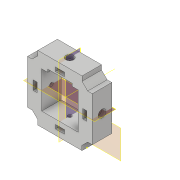
# Autodesk Inventor part: 30_Cube_Z_Focus_MGN_NEMA_Motorsupport_centered
Saved by Autodesk Inventor 2022 (Build 260153000, 153)
## iProperties
Created: 2019-07-01
Part Number: 30_Cube_Z_Focus_MGN_NEMA_Motorsupport_centered
Material: Generic
Document SubType Name: Modeling
Designer: diederichbenedict
Density: 1 g/cm^3
Appearance: Default
Author: diederichbenedict
Autodesk Inventor part; units mm, degrees
ref_plane "YZ Plane" through (0, 0, 0) normal (1, 0, 0) x (0, 1, 0)
ref_plane "XZ Plane" through (0, 0, 0) normal (0, 1, 0) x (-1, 0, 0)
ref_plane "XY Plane" through (0, 0, 0) normal (0, 0, 1) x (1, 0, 0)
ref_plane "Work Plane5" through (0, 0, 10) normal (0, 0, 1) x (1, 0, 0)
sketch "Sketch1" plane through (0, 0, 10) normal (0, 0, 1) x (1, 0, 0)
  line L0 (-4.0299, -0.3538) -> (-2.2322, 1.4439) construction
  arc A0 (-1.4439, 2.2322) -> (-2.2322, 1.4439) centre (-0.9299, 0.9299) ccw construction
  line L1 (-1.4439, 2.2322) -> (0.3538, 4.0299) construction
  line L2 (-37.8299, 42.8299) -> (-37.8299, 37.8299) construction
  line L3 (-37.8299, 37.8299) -> (-42.9208, 37.8299) construction
  line L4 (-37.8299, 42.2137) -> (-37.8299, 45.8299) construction
  line L5 (-37.8299, 45.8299) -> (-4.0299, 45.8299) construction
  line L6 (-4.0299, 45.8299) -> (-4.0299, 42.2137) construction
  line L7 (-4.0299, 4.0299) -> (0.3538, 4.0299) projected
  circle A1 centre (-20.9299, 20.9299) radius 17.5 projected
  line L8 (-20.9299, 58.9723) -> (17.1124, 20.9299) construction
  line L9 (17.1124, 20.9299) -> (-20.9299, -17.1124) construction
  line L10 (-20.9299, -17.1124) -> (-58.9723, 20.9299) construction
  line L11 (-58.9723, 20.9299) -> (-20.9299, 58.9723) construction
  line L12 (-20.9299, 58.9723) -> (-20.9299, -17.1124) construction
  line L13 (17.1124, 20.9299) -> (-58.9723, 20.9299) construction
  line L14 (-20.9299, 58.9723) -> (32.8701, 58.9723) construction
  line L15 (-43.4299, 43.4299) -> (1.5701, 43.4299) construction
  line L16 (1.5701, 43.4299) -> (1.5701, -1.5701) construction
  line L17 (1.5701, -1.5701) -> (-43.4299, -1.5701) construction
  line L18 (-43.4299, -1.5701) -> (-43.4299, 43.4299) construction
  line L19 (-43.4299, 43.4299) -> (1.5701, -1.5701) construction
  line L20 (1.5701, 43.4299) -> (-43.4299, -1.5701) construction
  line L21 (-43.4299, 5.3876) -> (-43.4299, 36.4723)
  line L22 (-43.4299, 36.4723) -> (-36.4723, 43.4299)
  line L23 (-36.4723, 43.4299) -> (-5.3876, 43.4299)
  line L24 (-5.3876, 43.4299) -> (1.5701, 36.4723)
  line L25 (1.5701, 36.4723) -> (1.5701, 5.3876)
  line L26 (1.5701, 5.3876) -> (-5.3876, -1.5701)
  line L27 (-5.3876, -1.5701) -> (-36.4723, -1.5701)
  line L28 (-36.4723, -1.5701) -> (-43.4299, 5.3876)
  line L29 (-4.0299, 42.2137) -> (-37.8299, 42.2137) projected
  line L30 (-4.0299, -0.3538) -> (-4.0299, 4.0299) projected
  circle A2 centre (-20.9299, 20.9299) radius 1.5
  line L31 (-10.9299, 10.9299) -> (-30.9299, 10.9299) construction
  line L32 (-30.9299, 10.9299) -> (-30.9299, 30.9299) construction
  line L33 (-30.9299, 30.9299) -> (-10.9299, 30.9299) construction
  line L34 (-10.9299, 30.9299) -> (-10.9299, 10.9299) construction
  line L35 (-10.9299, 10.9299) -> (-30.9299, 30.9299) construction
  line L36 (-30.9299, 10.9299) -> (-10.9299, 30.9299) construction
  circle A3 centre (-30.9299, 30.9299) radius 1.4
  circle A4 centre (-30.9299, 10.9299) radius 1.4
  circle A5 centre (-10.9299, 10.9299) radius 1.4
  line L37 (-45.8299, 37.8299) -> (-42.0723, 37.8299) construction
  line L38 (-42.1723, 37.7299) -> (-45.8299, 37.7299)
  line L39 (-45.8299, 37.7299) -> (-45.8299, 4.1299)
  line L40 (-45.8299, 4.1299) -> (-42.1723, 4.1299)
  line L41 (-42.1723, 4.1299) -> (-42.1723, 37.7299)
  line L42 (-45.8299, 4.0299) -> (-42.0723, 4.0299) construction
  line L43 (-45.8299, 37.8299) -> (-42.0723, 37.8299) projected
  line L44 (-37.7299, 45.8299) -> (-4.1299, 45.8299)
  line L45 (-4.1299, 45.8299) -> (-4.1299, 42.1723)
  line L46 (-4.1299, 42.1723) -> (-37.7299, 42.1723)
  line L47 (-37.7299, 42.1723) -> (-37.7299, 45.8299)
  line L48 (0.4701, 37.8299) -> (0.4701, 4.0299) construction
  line L49 (0.4701, 4.0299) -> (3.9701, 4.0299) construction
  line L50 (3.9701, 37.8299) -> (3.9701, 4.0299) construction
  line L51 (0.4701, 37.8299) -> (3.9701, 37.8299) construction
  line L52 (-45.8299, -3.9701) -> (-4.0299, -3.9701) construction
  line L53 (0.3124, 37.7299) -> (3.9701, 37.7299)
  line L54 (3.9701, 37.7299) -> (3.9701, 4.1299)
  line L55 (3.9701, 4.1299) -> (0.3124, 4.1299)
  line L56 (0.3124, 4.1299) -> (0.3124, 37.7299)
  line L57 (-4.1713, -0.3538) -> (-37.7299, -0.3538)
  line L58 (-37.7299, -0.3538) -> (-37.7299, -3.9701)
  line L59 (-37.7299, -3.9701) -> (-4.1713, -3.9701)
  line L60 (-4.1713, -3.9701) -> (-4.1713, -0.3538)
  point P0 (-37.8299, 4.0299)
  dimension "d18" = 53.8
  dimension "d19" = 45
  dimension "d20" = 53.8
  dimension "d21" = 45
  dimension "d22" = 45
  dimension "d30" = 20
  dimension "d31" = 20
  dimension "d32" = 2.8
  dimension "d33" = 2.8
  dimension "d34" = 2.8
  dimension "d35" = 3
  dimension "d36" = 0.1
  dimension "d37" = 0.1
  dimension "d38" = 0.1
  dimension "d39" = 0.1
  constraints: 86 end point, 21 point on line, 14 parallel, 8 perpendicular, 7 horizontal, 7 midpoint, 4 centre point, 4 coincident, 1 equal length
  measures "d18" distance of L8.start L8.end
  measures "d19" angle of L8 L14
  measures "d20" distance of L8.end L9.end
  measures "d21" distance of L16.end L17.end
  measures "d22" distance of L15.end L16.end
  measures "d30" distance of L32.end L33.end
  measures "d31" distance of L31.end L32.end
  measures "d32" diameter of A3
  measures "d33" diameter of A4
  measures "d34" diameter of A5
  measures "d35" diameter of A2
  measures "d36" distance between parallel lines of L38 L43
  measures "d37" distance between parallel lines of L40 L42
  measures "d38" distance between parallel lines of L45 L6
  measures "d39" distance between parallel lines of L4 L47
extrude "Extrusion1" add sketch "Sketch1" along normal blind 15 contours L30 L26 L57 L28 L41 L22 L46 L24 L56 L7 | L7 L26 L30 | L56 L24 L25 L26 | L26 L25 L24 L53 L54 L55 | L60 L59 L58 L57 L28 L27 L26 | L26 L27 L28 L57 | L46 L22 L29 L24 | L24 L29 L45 | L40 L39 L38 L22 L21 L28 | L28 L21 L22 L41 | L29 L22 L23 L24 | L24 L23 L22 L29 L47 L44 L45 | L47 L29 L22 | A1 | A2 | A3 | A4 | A5
sketch "Skizze4" plane through (0, 0, 25) normal (0, 0, 1) x (1, 0, 0)
  line L0 (-37.7299, 42.1723) -> (-42.1723, 37.7299) projected
  line L1 (-42.1723, 37.7299) -> (-45.8299, 37.7299) projected
  line L2 (-45.8299, 37.7299) -> (-45.8299, 4.1299) construction
  line L3 (-45.8299, 4.1299) -> (-42.1723, 4.1299) projected
  line L4 (-42.1723, 4.1299) -> (-37.6885, -0.3538) projected
  line L5 (-37.6885, -0.3538) -> (-37.7299, -0.3538) projected
  line L6 (-37.7299, -0.3538) -> (-37.7299, -3.9701) projected
  line L7 (-37.7299, -3.9701) -> (-4.1713, -3.9701) construction
  line L8 (-4.1713, -3.9701) -> (-4.1713, -0.3538) projected
  line L9 (-4.1713, -0.3538) -> (0.3124, 4.1299) projected
  line L10 (0.3124, 4.1299) -> (3.9701, 4.1299) projected
  line L11 (3.9701, 4.1299) -> (3.9701, 37.7299) construction
  line L12 (3.9701, 37.7299) -> (0.3124, 37.7299) projected
  line L13 (0.3124, 37.7299) -> (-4.1299, 42.1723) projected
  line L14 (-4.1299, 42.1723) -> (-4.1299, 45.8299) projected
  line L15 (-4.1299, 45.8299) -> (-37.7299, 45.8299) construction
  line L16 (-37.7299, 45.8299) -> (-37.7299, 42.1723) projected
  line L17 (-37.9299, 46.0299) -> (-3.9299, 46.0299) construction
  line L18 (-3.9299, 46.0299) -> (-3.9299, 42.2551)
  line L19 (-3.9299, 42.2551) -> (0.3953, 37.9299)
  line L20 (0.3953, 37.9299) -> (4.1701, 37.9299)
  line L21 (4.1701, 37.9299) -> (4.1701, 3.9299) construction
  line L22 (4.1701, 3.9299) -> (0.3953, 3.9299)
  line L23 (0.3953, 3.9299) -> (-3.9713, -0.4367)
  line L24 (-3.9713, -0.4367) -> (-3.9713, -4.1701)
  line L25 (-3.9713, -4.1701) -> (-37.9299, -4.1701) construction
  line L26 (-37.9299, -4.1701) -> (-37.9299, -0.3953)
  line L27 (-37.9299, -0.3953) -> (-42.2551, 3.9299)
  line L28 (-42.2551, 3.9299) -> (-46.0299, 3.9299)
  line L29 (-46.0299, 3.9299) -> (-46.0299, 37.9299) construction
  line L30 (-46.0299, 37.9299) -> (-42.2551, 37.9299)
  line L31 (-42.2551, 37.9299) -> (-37.9299, 42.2551)
  line L32 (-37.9299, 42.2551) -> (-37.9299, 46.0299)
  line L33 (-45.8299, 37.7299) -> (-45.8299, 37.9299)
  line L34 (-4.1299, 45.8299) -> (-37.7299, 45.8299) projected
  line L35 (-37.7299, 45.8299) -> (-37.9299, 45.8299)
  line L36 (-4.1299, 45.8299) -> (-3.9299, 45.8299)
  line L37 (3.9701, 37.7299) -> (3.9701, 37.9299)
  line L38 (3.9701, 4.1299) -> (3.9701, 37.7299) projected
  line L39 (3.9701, 4.1299) -> (3.9701, 3.9299)
  line L40 (-4.1713, -3.9701) -> (-3.9713, -3.9701)
  line L41 (-37.7299, -3.9701) -> (-37.9299, -3.9701)
  line L42 (-45.8299, 4.1299) -> (-45.8299, 3.9299)
  point P0 (0, 0)
  dimension "d40" = 0.2
  constraints: 48 end point, 12 point on line, 4 perpendicular, 15 other
  measures "d40" distance between parallel lines of L15 L17
extrude "IM_offset" add sketch "Skizze4" against normal up to surface (15 mm away)
sketch "Sketch29" plane through (0, 0, 10) normal (0, 0, -1) x (-1, 0, 0)
  line L0 (30.9299, 15.9299) -> (30.9299, 25.9299)
  line L1 (25.9299, 30.9299) -> (15.8299, 30.9299)
  line L2 (10.9299, 29.4299) -> (10.9299, 12.4299)
  line L3 (29.4299, 10.9299) -> (12.4299, 10.9299)
  line L4 (10.9299, 10.9299) -> (30.9299, 10.9299) construction
  line L5 (30.9299, 10.9299) -> (30.9299, 30.9299)
  line L6 (30.9299, 30.9299) -> (10.9299, 30.9299)
  line L7 (10.9299, 30.9299) -> (10.9299, 10.9299)
  line L8 (10.8299, 10.8299) -> (31.0299, 10.8299)
  line L9 (31.0299, 10.8299) -> (31.0299, 31.0299)
  line L10 (31.0299, 31.0299) -> (10.8299, 31.0299)
  line L11 (10.8299, 31.0299) -> (10.8299, 10.8299)
  circle A0 centre (20.9299, 20.9299) radius 11
  line L12 (13.0299, 34.4299) -> (28.8299, 34.4299)
  line L13 (6.9299, 12.5299) -> (6.9299, 29.3299)
  line L14 (34.9299, 9.4299) -> (34.9299, 32.4299)
  line L15 (29.3299, 6.9299) -> (12.5299, 6.9299)
  line L16 (12.5299, 34.9299) -> (29.3299, 34.9299)
  line L17 (34.9299, 6.9299) -> (6.9299, 6.9299)
  line L18 (6.9299, 6.9299) -> (6.9299, 34.9299)
  line L19 (6.9299, 34.9299) -> (34.9299, 34.9299)
  line L20 (34.9299, 34.9299) -> (34.9299, 6.9299)
  line L21 (34.9299, 6.9299) -> (6.9299, 34.9299) construction
  line L22 (6.9299, 6.9299) -> (34.9299, 34.9299) construction
  line L23 (35.0299, 35.0299) -> (6.8299, 35.0299)
  line L24 (6.8299, 35.0299) -> (6.8299, 6.8299)
  line L25 (6.8299, 6.8299) -> (35.0299, 6.8299)
  line L26 (35.0299, 6.8299) -> (35.0299, 35.0299)
  point P0 (0, 0)
  dimension "d188" = 0.1
  dimension "d189" = 0.1
  constraints: 54 end point, 8 parallel, 7 horizontal, 4 perpendicular, 4 vertical, 2 midpoint, 1 centre point, 26 other
  measures "d188" distance between parallel lines of L7 L11
  measures "d189" distance between parallel lines of L19 L23
extrude "Extrusion23" cut sketch "Sketch29" against normal through all contours A0 L3 L2 L1 L0 | A0 L9 L8 | L0 A0 L9 | A0 L1 L6 L5 L0 | L0 L5 L6 L1 A0 L10 L9 | A0 L8 L3 | L9 A0 | L1 A0 L10 | A0 L8 L11 | A0 L8 | A0 L2 L7 L6 L1 | L1 L6 L7 L2 A0 L11 L10 | L10 A0 | A0 L11 L2 | A0 L11 | L13 L18 L19 L16 L20 L14 L17 L15 | L26 L25 L24 L23
sketch "Sketch30" plane through (-45.8299, 0, 10) normal (-1, 0, 0) x (0, 0, 1)
  line L0 (35.0799, 45.8299) -> (6.8799, 45.8299)
  line L1 (0, 3.9299) -> (0, 37.9299) projected
  line L2 (15, 3.9299) -> (0, 3.9299) projected
  line L3 (15, 37.9299) -> (15, 3.9299) projected
  line L4 (15, 37.9299) -> (0, 37.9299) projected
  circle A0 centre (7.5, 20.9299) radius 1.7201
  point P0 (-10, 0)
  constraints: 2 end point, 1 centre point, 1 horizontal
ref_plane "Arbeitsebene7" through (-20.9299, 3.9299, 10) normal (-1, 0, 0) x (0, 0, 1)
ref_plane "Arbeitsebene8" through (-37.9299, 20.9299, 10) normal (0, 1, 0) x (1, 0, 0)
ref_plane "Arbeitsebene9" through (-20.9299, 3.9299, 10) normal (-1, 0, 0) x (0, 0, 1)
ref_plane "Arbeitsebene10" through (-37.9299, 20.9299, 10) normal (0, -1, 0) x (1, 0, 0)
hole "Bohrung2" at (-45.8299, 20.9299, 17.5) direction (1, 0, 0) diameter 2.8 end through all counterbore diameter 6 counterbore depth 3
pattern_circular "Runde Anordnung2" count 4 over 360 about axis through (-20.9299, 20.9299, 10) along (0, 0, 1) of "Bohrung2"
ref_plane "Arbeitsebene11" through (-20.9299, 3.9299, 10) normal (1, 0, 0) x (0, 0, -1)
ref_plane "Arbeitsebene12" through (-37.9299, 20.9299, 10) normal (0, 1, 0) x (1, 0, 0)
sketch "Sketch31" plane through (0, 0, 25) normal (0, 0, 1) x (1, 0, 0)
  point P0 (0, 0)
sketch "Sketch32" plane through (0, 0, 25) normal (0, 0, 1) x (1, 0, 0)
  line L0 (-6.8299, 6.8299) -> (-35.0299, 6.8299) projected
  line L1 (-35.0299, 6.8299) -> (-35.0299, 35.0299) projected
  line L2 (-35.0299, 35.0299) -> (-6.8299, 35.0299) projected
  line L3 (-6.8299, 35.0299) -> (-6.8299, 6.8299) projected
  line L4 (3.9701, 3.9299) -> (3.9701, 37.9299) projected
  line L5 (3.9701, 37.9299) -> (0.3953, 37.9299) projected
  line L6 (0.3953, 37.9299) -> (-3.9299, 42.2551) projected
  line L7 (-3.9299, 42.2551) -> (-3.9299, 45.8299) projected
  line L8 (-3.9299, 45.8299) -> (-37.9299, 45.8299) projected
  line L9 (-37.9299, 45.8299) -> (-37.9299, 42.2551) projected
  line L10 (-37.9299, 42.2551) -> (-42.2551, 37.9299) projected
  line L11 (-42.2551, 37.9299) -> (-45.8299, 37.9299) projected
  line L12 (-45.8299, 37.9299) -> (-45.8299, 3.9299) projected
  line L13 (-42.2551, 3.9299) -> (-45.8299, 3.9299) projected
  line L14 (-37.9299, -0.3953) -> (-42.2551, 3.9299) projected
  line L15 (-37.9299, -3.9701) -> (-37.9299, -0.3953) projected
  line L16 (-3.9713, -3.9701) -> (-37.9299, -3.9701) projected
  line L17 (-3.9713, -3.9701) -> (-3.9713, -0.4367) projected
  line L18 (-3.9713, -0.4367) -> (0.3953, 3.9299) projected
  line L19 (0.3953, 3.9299) -> (3.9701, 3.9299) projected
  line L20 (-22.3299, 42.8299) -> (-22.3299, 35.0299) projected
  line L21 (-19.5299, 42.8299) -> (-19.5299, 35.0299) projected
  line L22 (0.9701, 22.3299) -> (-6.8299, 22.3299) projected
  line L23 (0.9701, 19.5299) -> (-6.8299, 19.5299) projected
  line L24 (-19.5299, 6.8299) -> (-19.5299, -0.9701) projected
  line L25 (-22.3299, 6.8299) -> (-22.3299, -0.9701) projected
  line L26 (-35.0299, 19.5299) -> (-42.8299, 19.5299) projected
  line L27 (-35.0299, 22.3299) -> (-42.8299, 22.3299) projected
  line L28 (-41.5925, 24.4299) -> (-38.5925, 24.4299)
  line L29 (-38.5925, 24.4299) -> (-38.5925, 17.4299)
  line L30 (-38.5925, 17.4299) -> (-41.5925, 17.4299)
  line L31 (-41.5925, 17.4299) -> (-41.5925, 24.4299)
  line L32 (-41.5925, 24.4299) -> (-38.5925, 17.4299) construction
  line L33 (-38.5925, 24.4299) -> (-41.5925, 17.4299) construction
  point P0 (0, 0)
  point P1 (-40.0925, 20.9299)
  dimension "d190" = 3
  dimension "d191" = 7
  constraints: 12 end point, 2 midpoint, 2 parallel, 1 horizontal, 1 perpendicular
  measures "d190" distance of L29.end L30.end
  measures "d191" distance of L28.end L29.end
extrude "Extrusion25" cut sketch "Sketch32" against normal through all contours L29 L30 L31 L26 | L26 L31 L27 L29 | L27 L31 L28 L29
pattern_circular "Circular Pattern3" count 4 over 360 about axis through (-20.9299, 20.9299, 10) along (0, 0, 1) of "Extrusion25"
sketch "Sketch33" plane through (0, 0, 25) normal (0, 0, 1) x (1, 0, 0)
  line L0 (-24.4299, 38.5925) -> (-24.4299, 41.5925) projected
  line L1 (-24.4299, 41.5925) -> (-17.4299, 41.5925) projected
  line L2 (-17.4299, 41.5925) -> (-17.4299, 38.5925) projected
  line L3 (-17.4299, 38.5925) -> (-24.4299, 38.5925) projected
  line L4 (-3.2673, 24.4299) -> (-0.2673, 24.4299) projected
  line L5 (-0.2673, 24.4299) -> (-0.2673, 17.4299) projected
  line L6 (-0.2673, 17.4299) -> (-3.2673, 17.4299) projected
  line L7 (-3.2673, 17.4299) -> (-3.2673, 24.4299) projected
  line L8 (-17.4299, 3.2673) -> (-17.4299, 0.2673) projected
  line L9 (-17.4299, 0.2673) -> (-24.4299, 0.2673) projected
  line L10 (-24.4299, 0.2673) -> (-24.4299, 3.2673) projected
  line L11 (-24.4299, 3.2673) -> (-17.4299, 3.2673) projected
  line L12 (-41.5925, 24.4299) -> (-38.5925, 24.4299) projected
  line L13 (-38.5925, 24.4299) -> (-38.5925, 17.4299) projected
  line L14 (-38.5925, 17.4299) -> (-41.5925, 17.4299) projected
  line L15 (-41.5925, 17.4299) -> (-41.5925, 24.4299) projected
  line L16 (-6.8299, 6.8299) -> (-35.0299, 6.8299) projected
  line L17 (-35.0299, 6.8299) -> (-35.0299, 35.0299) projected
  line L18 (-35.0299, 35.0299) -> (-6.8299, 35.0299) projected
  line L19 (-6.8299, 35.0299) -> (-6.8299, 6.8299) projected
  line L20 (3.9701, 3.9299) -> (3.9701, 37.9299) projected
  line L21 (3.9701, 37.9299) -> (0.3953, 37.9299) projected
  line L22 (0.3953, 37.9299) -> (-3.9299, 42.2551) projected
  line L23 (-3.9299, 42.2551) -> (-3.9299, 45.8299) projected
  line L24 (-3.9299, 45.8299) -> (-37.9299, 45.8299) projected
  line L25 (-37.9299, 45.8299) -> (-37.9299, 42.2551) projected
  line L26 (-37.9299, 42.2551) -> (-42.2551, 37.9299) projected
  line L27 (-42.2551, 37.9299) -> (-45.8299, 37.9299) projected
  line L28 (-45.8299, 37.9299) -> (-45.8299, 3.9299) projected
  line L29 (-42.2551, 3.9299) -> (-45.8299, 3.9299) projected
  line L30 (-37.9299, -0.3953) -> (-42.2551, 3.9299) projected
  line L31 (-37.9299, -3.9701) -> (-37.9299, -0.3953) projected
  line L32 (-3.9713, -3.9701) -> (-37.9299, -3.9701) projected
  line L33 (-3.9713, -3.9701) -> (-3.9713, -0.4367) projected
  line L34 (-3.9713, -0.4367) -> (0.3953, 3.9299) projected
  line L35 (0.3953, 3.9299) -> (3.9701, 3.9299) projected
  line L36 (-11.4941, 32.8797) -> (-30.3658, 32.8797)
  line L37 (-30.3658, 32.8797) -> (-30.3658, 37.1801)
  line L38 (-30.3658, 37.1801) -> (-11.4941, 37.1801)
  line L39 (-11.4941, 37.1801) -> (-11.4941, 32.8797)
  line L40 (-6.8299, 35.0299) -> (-35.0299, 35.0299) projected
  line L41 (-11.4941, 32.8797) -> (-30.3658, 37.1801) construction
  line L42 (-30.3658, 32.8797) -> (-11.4941, 37.1801) construction
  point P0 (0, 0)
  point P1 (-20.9299, 35.0299)
  constraints: 12 end point, 3 midpoint, 2 parallel, 1 horizontal, 1 perpendicular
extrude "Extrusion26" cut sketch "Sketch33" against normal through all contours L39 L36 L37 L18 | L18 L37 L38 L39
body "Solid1"
